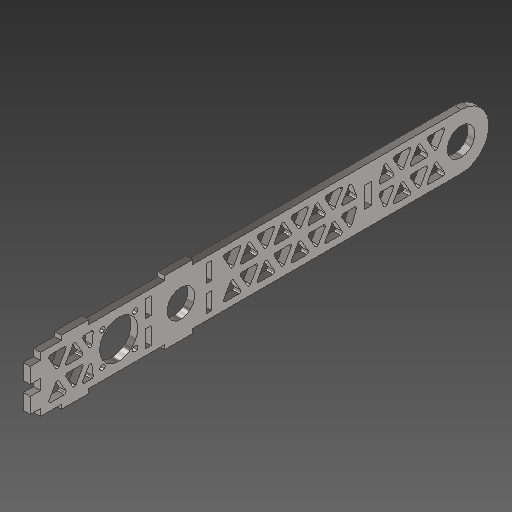
# Autodesk Inventor part: NeckFrame_02
Saved by Autodesk Inventor 2021 (Build 250183000, 183)
## iProperties
Created: 2021-03-08
Part Number: NeckFrame_02
Material: Steel, High Strength, Low Alloy
Document SubType Name: Modeling
Designer: M3rob
Density: 7.85 g/cm^3
Appearance: Steel - Polished
Mass: 5898.96 g
Surface Area: 1928.08 cm^2
Volume: 751.46 cm^3
Author: M3rob
Autodesk Inventor part; units mm, degrees
ref_plane "YZ Plane" through (0, 0, 0) normal (1, 0, 0) x (0, 1, 0)
ref_plane "XZ Plane" through (0, 0, 0) normal (0, 1, 0) x (-1, 0, 0)
ref_plane "XY Plane" through (0, 0, 0) normal (0, 0, 1) x (1, 0, 0)
sketch "Sketch1" plane through (0, 0, 0) normal (1, 0, 0) x (0, 1, 0)
  line L0 (50.8, 410.849) -> (38.1, 410.849)
  line L1 (-50.8, 410.849) -> (-50.8, 372.749)
  arc A0 (-50.8, -360.049) -> (50.8, -360.049) centre (0, -360.049) ccw
  line L2 (50.8, -360.049) -> (50.8, 132.084)
  line L3 (50.8, -360.049) -> (50.8, -410.849) construction
  line L4 (50.8, -410.849) -> (-50.8, -410.849) construction
  line L5 (-50.8, -410.849) -> (-50.8, -360.049) construction
  line L6 (0, 410.849) -> (0, -410.849) construction
  line L7 (38.1, 410.849) -> (38.1, 429.899)
  line L8 (38.1, 429.899) -> (9.525, 429.899)
  line L9 (9.525, 429.899) -> (9.525, 410.849)
  line L10 (-9.525, 410.849) -> (-9.525, 429.899)
  line L11 (-9.525, 429.899) -> (-38.1, 429.899)
  line L12 (-38.1, 429.899) -> (-38.1, 410.849)
  line L13 (9.525, 410.849) -> (-9.525, 410.849)
  line L14 (38.1, 410.849) -> (9.525, 410.849) construction
  line L15 (-9.525, 410.849) -> (-38.1, 410.849) construction
  line L16 (-38.1, 410.849) -> (-50.8, 410.849)
  line L17 (39.6875, 106.684) -> (7.9375, 106.684)
  line L18 (7.9375, 106.684) -> (7.9375, 97.159)
  line L19 (7.9375, 97.159) -> (39.6875, 97.159)
  line L20 (39.6875, 97.159) -> (39.6875, 106.684)
  line L21 (39.6875, 106.684) -> (7.9375, 97.159) construction
  line L22 (7.9375, 106.684) -> (39.6875, 97.159) construction
  line L23 (-39.6875, 106.684) -> (-7.9375, 106.684)
  line L24 (-7.9375, 106.684) -> (-7.9375, 97.159)
  line L25 (-7.9375, 97.159) -> (-39.6875, 97.159)
  line L26 (-39.6875, 97.159) -> (-39.6875, 106.684)
  line L27 (-39.6875, 106.684) -> (-7.9375, 97.159) construction
  line L28 (-7.9375, 106.684) -> (-39.6875, 97.159) construction
  line L29 (50.8, 372.749) -> (58.7375, 372.749)
  line L30 (58.7375, 372.749) -> (58.7375, 321.949)
  line L31 (58.7375, 321.949) -> (50.8, 321.949)
  line L32 (50.8, 182.884) -> (58.7375, 182.884)
  line L33 (58.7375, 182.884) -> (58.7375, 132.084)
  line L34 (58.7375, 132.084) -> (50.8, 132.084)
  line L35 (-50.8, 132.084) -> (-58.7375, 132.084)
  line L36 (-58.7375, 132.084) -> (-58.7375, 182.884)
  line L37 (-58.7375, 182.884) -> (-50.8, 182.884)
  line L38 (7.9375, 217.809) -> (39.6875, 217.809)
  line L39 (39.6875, 217.809) -> (39.6875, 208.284)
  line L40 (39.6875, 208.284) -> (7.9375, 208.284)
  line L41 (7.9375, 208.284) -> (7.9375, 217.809)
  line L42 (7.9375, 217.809) -> (39.6875, 208.284) construction
  line L43 (39.6875, 217.809) -> (7.9375, 208.284) construction
  line L44 (-39.6875, 217.809) -> (-7.9375, 217.809)
  line L45 (-7.9375, 217.809) -> (-7.9375, 208.284)
  line L46 (-7.9375, 208.284) -> (-39.6875, 208.284)
  line L47 (-39.6875, 208.284) -> (-39.6875, 217.809)
  line L48 (-39.6875, 217.809) -> (-7.9375, 208.284) construction
  line L49 (-7.9375, 217.809) -> (-39.6875, 208.284) construction
  line L50 (23.8125, 213.0465) -> (23.8125, 101.9215) construction
  line L51 (-50.8, 372.749) -> (-58.7375, 372.749)
  line L52 (-58.7375, 372.749) -> (-58.7375, 321.949)
  line L53 (-58.7375, 321.949) -> (-50.8, 321.949)
  line L54 (50.8, 321.949) -> (50.8, 372.749) construction
  line L55 (50.8, 372.749) -> (50.8, 410.849) construction
  line L56 (-50.8, 321.949) -> (-50.8, 398.5427)
  line L57 (-50.8, 372.749) -> (-50.8, 321.949) construction
  line L58 (-50.8, 182.884) -> (-50.8, 132.084) construction
  line L59 (-50.8, 132.084) -> (-50.8, -360.049)
  line L60 (50.8, 182.884) -> (50.8, 385.0553)
  line L61 (50.8, 132.084) -> (50.8, 182.884) construction
  line L62 (50.8, 398.5427) -> (41.275, 398.5427)
  line L63 (41.275, 398.5427) -> (41.275, 401.324)
  line L64 (41.275, 401.324) -> (33.3375, 401.324)
  line L65 (33.3375, 401.324) -> (33.3375, 398.5427)
  line L66 (33.3375, 398.5427) -> (30.1625, 398.5427)
  line L67 (30.1625, 398.5427) -> (30.1625, 385.0553)
  line L68 (30.1625, 385.0553) -> (33.3375, 385.0553)
  line L69 (33.3375, 385.0553) -> (33.3375, 382.274)
  line L70 (33.3375, 382.274) -> (41.275, 382.274)
  line L71 (41.275, 382.274) -> (41.275, 385.0553)
  line L72 (41.275, 385.0553) -> (50.8, 385.0553)
  line L73 (30.1625, 391.799) -> (50.8, 391.799) construction
  line L74 (-50.8, 398.5427) -> (-41.275, 398.5427)
  line L75 (-41.275, 398.5427) -> (-41.275, 401.324)
  line L76 (-41.275, 401.324) -> (-33.3375, 401.324)
  line L77 (-33.3375, 401.324) -> (-33.3375, 398.5427)
  line L78 (-33.3375, 398.5427) -> (-30.1625, 398.5427)
  line L79 (-30.1625, 398.5427) -> (-30.1625, 385.0553)
  line L80 (-30.1625, 385.0553) -> (-33.3375, 385.0553)
  line L81 (-33.3375, 385.0553) -> (-33.3375, 382.274)
  line L82 (-33.3375, 382.274) -> (-41.275, 382.274)
  line L83 (-41.275, 382.274) -> (-41.275, 385.0553)
  line L84 (-50.8, 385.0553) -> (-41.275, 385.0553)
  line L85 (50.8, 398.5427) -> (50.8, 321.949) construction
  line L86 (50.8, 385.0553) -> (50.8, 398.5427)
  line L87 (-50.8, 385.0553) -> (-50.8, 182.884)
  line L88 (-50.8, 398.5427) -> (-50.8, 385.0553) construction
  circle A1 centre (0, 267.339) radius 35.052
  circle A2 centre (0, 153.492) radius 25.4
  line L89 (50.8, 398.5427) -> (50.8, 410.849)
  line L90 (50.8, 385.0553) -> (50.8, 372.749)
  arc A3 (-32.4225, 153.492) -> (32.4225, 153.492) centre (0, 153.492) ccw
  circle A4 centre (0, -360.049) radius 25.4
  arc A5 (-62.6143, -356.6081) -> (62.6143, -356.6081) centre (0, -360.049) ccw
  point P0 (0, 0)
  point P1 (0, 0)
  point P2 (-23.8125, 101.9215)
  point P3 (23.8125, 213.0465)
  point P4 (-23.8125, 213.0465)
  point P5 (23.8125, 429.899)
  point P6 (58.7375, 157.484)
  point P7 (23.8125, 157.484)
  point P8 (23.8125, 391.799)
  point P9 (-30.1625, 391.799)
  point P10 (-50.8, 372.749)
  point P11 (-50.8, 372.749)
  dimension "d0" = 101.6
  dimension "d3" = 19.05
  dimension "d4" = 12.7
  dimension "d5" = 19.05
  dimension "d6" = 9.525
  dimension "d8" = 7.9375
  dimension "d9" = 50.8
  dimension "d12" = 31.75
  dimension "d13" = 38.1
  dimension "d14" = 9.525
  dimension "d15" = 7.9375
  dimension "d16" = 3.175
  dimension "d17" = 19.05
  dimension "d18" = 13.4874
  dimension "d23" = 143.51
  dimension "d24" = 70.104
  dimension "d25" = 50.8
  dimension "d26" = 19.05
  dimension "d39" = 50.8
  dimension "d86" = 101.6
  dimension "d92" = 193.04
  constraints: 182 end point, 100 perpendicular, 32 point on line, 18 midpoint, 15 equal length, 15 tangent, 14 horizontal, 10 vertical, 9 parallel, 6 centre point, 6 point on circle, 5 horizontal alignment, 3 concentric, 3 vertical alignment, 1 coincident, 1 collinear, 15 other
  measures "d0" distance of L0.start L1.start
  measures "d3" diameter of L9 L6
  measures "d4" distance from line of L0.start L7
  measures "d5" distance of L0.end L7.end
  measures "d6" distance of L19.end L17.start
  measures "d8" distance of L33.end L2.end
  measures "d9" distance of L32.end L33.end
  measures "d12" distance of L18.end L19.end
  measures "d13" distance from line of L29 L0.start
  measures "d14" distance of L71.end L60.end
  measures "d15" distance of L69.end L70.end
  measures "d16" distance of L67.end L68.end
  measures "d17" distance of L69.end L64.end
  measures "d18" distance between parallel lines of L72 L62
  measures "d23" distance from line of L14 A1.centre
  measures "d24" diameter of A1
  measures "d25" diameter of A2
  measures "d26" distance from line of L0 L73.end
  measures "d39" diameter of A4
  measures "d86" distance between parallel lines of L40 L17
  measures "d92" distance between parallel lines of L38 L0
extrude "Extrusion1" add sketch "Sketch1" along normal mid plane 12.7
sketch "Sketch3" plane through (6.35, 0, 0) normal (1, 0, 0) x (0, 0, -1)
  circle A0 centre (-267.339, 0) radius 34.925 construction
  line L0 (-224.159, 43.18) -> (-310.519, 43.18) construction
  line L1 (-310.519, 43.18) -> (-267.339, 0) construction
  line L2 (-310.519, -43.18) -> (-224.159, -43.18) construction
  line L3 (-267.339, 0) -> (-224.159, -43.18) construction
  line L4 (-224.159, -43.18) -> (-224.159, 43.18) construction
  line L5 (-224.159, 43.18) -> (-267.339, 0) construction
  line L6 (-310.519, 43.18) -> (-310.519, -43.18) construction
  line L7 (-267.339, 0) -> (-310.519, -43.18) construction
  circle A1 centre (-297.1803, 29.8414) radius 7.2771 construction
  circle A2 centre (-297.1803, -29.8414) radius 7.2771 construction
  circle A3 centre (-237.4976, -29.8414) radius 7.2771 construction
  circle A4 centre (-237.4976, 29.8414) radius 7.2771 construction
  circle A5 centre (-267.339, 25.019) radius 2.3813
  circle A6 centre (-292.358, 0) radius 2.3813
  circle A7 centre (-267.339, -25.019) radius 2.3813
  circle A8 centre (-242.32, 0) radius 2.3813
  circle A9 centre (-267.339, 0) radius 17.5768
  circle A10 centre (-267.339, 0) radius 35.052 projected
  dimension "d29" = 69.85
  dimension "d30" = 14.5542
  dimension "d31" = 360
  constraints: 16 end point, 10 centre point, 5 coincident, 2 collinear, 2 point on line, 1 perpendicular, 1 tangent, 13 other
  measures "d29" diameter of A0
  measures "d30" diameter of A1
hole "Hole1" at (6.35, 29.8414, 297.1803) at (6.35, 29.8414, 237.4976) at (6.35, -29.8414, 237.4976) at (6.35, -29.8414, 297.1803) direction (-1, 0, 0) diameter 9.779 end through all
sketch "Sketch4" plane through (6.35, 0, 0) normal (1, 0, 0) x (0, 0, -1)
  circle A0 centre (-358.4422, -15.0646) radius 101.6
  circle A1 centre (360.049, 0) radius 25.4
  line L0 (-90.809, 4.7625) -> (-90.809, 36.5125)
  circle A2 centre (360.049, 0) radius 406.4
  line L1 (-399.5955, -107.9568) -> (195.4357, -371.5689)
  line L2 (195.4357, -371.5689) -> (195.4357, 371.5689)
  line L3 (-65.409, -68.2625) -> (-65.409, 65.0875)
  circle A3 centre (360.049, 0) radius 25.4 projected
  line L4 (195.4357, 0) -> (182.7357, 0)
  line L5 (182.7357, 0) -> (182.7357, 19.05)
  line L6 (182.7357, 19.05) -> (195.4357, 19.05)
  line L7 (195.4357, 19.05) -> (195.4357, 0)
  line L8 (195.4357, 0) -> (182.7357, 0)
  line L9 (182.7357, 0) -> (182.7357, -19.05)
  line L10 (182.7357, -19.05) -> (195.4357, -19.05)
  line L11 (195.4357, -19.05) -> (195.4357, 0)
  point P0 (0, 0)
  point P1 (195.4357, -19.05)
  point P2 (195.4357, 19.05)
  dimension "d40" = 812.8
  dimension "d41" = 12.7
  dimension "d42" = 19.05
  dimension "d43" = 12.7
  dimension "d44" = 19.05
  dimension "d47" = 164.6133
  constraints: 24 end point, 5 parallel, 2 centre point, 2 coincident, 2 horizontal, 2 perpendicular, 2 point on circle, 1 midpoint, 1 tangent, 1 vertical, 4 other
  measures "d40" diameter of A2
  measures "d41" distance of L5.end L6.end
  measures "d42" distance of L4.end L5.end
  measures "d43" distance of L10.end L9.end
  measures "d44" distance of L9.end L8.end
  measures "d47" distance of A1.centre L4.start
extrude "Extrusion2" cut sketch "Sketch4" against normal through all contours L10 L9 L4 L2 | L2 L4 L5 L6
sketch "Sketch5" plane through (6.35, 0, 0) normal (1, 0, 0) x (0, 0, -1)
  line L0 (195.4357, -19.05) -> (182.7357, -19.05) construction
  line L1 (182.7357, -19.05) -> (182.7357, 19.05) construction
  line L2 (182.7357, 19.05) -> (195.4357, 19.05) construction
  line L3 (195.4357, 19.05) -> (195.4357, -19.05) construction
  circle A0 centre (-237.4976, -29.8414) radius 4.8895 construction
  circle A1 centre (-297.1803, 29.8414) radius 4.8895 construction
  circle A2 centre (-237.4976, 29.8414) radius 4.8895 construction
  circle A3 centre (-297.1803, -29.8414) radius 4.8895 construction
  line L4 (-410.849, -50.8) -> (-372.749, -50.8) construction
  line L5 (-372.749, -50.8) -> (-372.749, -58.7375) construction
  line L6 (-372.749, -58.7375) -> (-321.949, -58.7375) construction
  line L7 (-321.949, -58.7375) -> (-321.949, -50.8) construction
  line L8 (-321.949, -50.8) -> (-182.884, -50.8) construction
  line L9 (-182.884, -50.8) -> (-182.884, -58.7375) construction
  line L10 (-182.884, -58.7375) -> (-132.084, -58.7375) construction
  line L11 (-132.084, -58.7375) -> (-132.084, -50.8) construction
  line L12 (-132.084, -50.8) -> (360.049, -50.8) construction
  arc A4 (360.049, -50.8) -> (360.049, 50.8) centre (360.049, 0) ccw construction
  line L13 (360.049, 50.8) -> (-132.084, 50.8) construction
  line L14 (-132.084, 50.8) -> (-132.084, 58.7375) construction
  line L15 (-132.084, 58.7375) -> (-182.884, 58.7375) construction
  line L16 (-182.884, 58.7375) -> (-182.884, 50.8) construction
  line L17 (-182.884, 50.8) -> (-321.949, 50.8) construction
  line L18 (-321.949, 50.8) -> (-321.949, 58.7375) construction
  line L19 (-321.949, 58.7375) -> (-372.749, 58.7375) construction
  line L20 (-372.749, 58.7375) -> (-372.749, 50.8) construction
  line L21 (-372.749, 50.8) -> (-410.849, 50.8) construction
  line L22 (-410.849, 50.8) -> (-410.849, 38.1) construction
  line L23 (-410.849, 38.1) -> (-429.899, 38.1) construction
  line L24 (-429.899, 38.1) -> (-429.899, 9.525) construction
  line L25 (-429.899, 9.525) -> (-410.849, 9.525) construction
  line L26 (-410.849, 9.525) -> (-410.849, -9.525) construction
  line L27 (-410.849, -9.525) -> (-429.899, -9.525) construction
  line L28 (-429.899, -9.525) -> (-429.899, -38.1) construction
  line L29 (-429.899, -38.1) -> (-410.849, -38.1) construction
  line L30 (-410.849, -38.1) -> (-410.849, -50.8) construction
  circle A5 centre (-267.339, 0) radius 35.052 construction
  circle A6 centre (360.049, 0) radius 25.4 construction
  circle A7 centre (-153.492, 0) radius 25.4 construction
  line L31 (-217.809, -39.6875) -> (-217.809, -7.9375) construction
  line L32 (-217.809, -7.9375) -> (-208.284, -7.9375) construction
  line L33 (-208.284, -7.9375) -> (-208.284, -39.6875) construction
  line L34 (-208.284, -39.6875) -> (-217.809, -39.6875) construction
  line L35 (-217.809, 7.9375) -> (-217.809, 39.6875) construction
  line L36 (-217.809, 39.6875) -> (-208.284, 39.6875) construction
  line L37 (-208.284, 39.6875) -> (-208.284, 7.9375) construction
  line L38 (-208.284, 7.9375) -> (-217.809, 7.9375) construction
  line L39 (-106.684, -39.6875) -> (-106.684, -7.9375) construction
  line L40 (-106.684, -7.9375) -> (-97.159, -7.9375) construction
  line L41 (-97.159, -7.9375) -> (-97.159, -39.6875) construction
  line L42 (-97.159, -39.6875) -> (-106.684, -39.6875) construction
  line L43 (-106.684, 39.6875) -> (-97.159, 39.6875) construction
  line L44 (-97.159, 39.6875) -> (-97.159, 7.9375) construction
  line L45 (-97.159, 7.9375) -> (-106.684, 7.9375) construction
  line L46 (-106.684, 7.9375) -> (-106.684, 39.6875) construction
  line L47 (-140.0215, 38.1) -> (360.049, 38.1) construction
  arc A8 (360.049, -38.1) -> (360.049, 38.1) centre (360.049, 0) ccw construction
  line L48 (360.049, -38.1) -> (-140.0215, -38.1) construction
  line L49 (-140.0215, -38.1) -> (-140.0215, -46.0375) construction
  line L50 (-140.0215, -46.0375) -> (-165.4215, -46.0375) construction
  line L51 (-165.4215, -46.0375) -> (-165.4215, -38.1) construction
  line L52 (-165.4215, -38.1) -> (-334.649, -38.1) construction
  line L53 (-334.649, -38.1) -> (-334.649, -46.0375) construction
  line L54 (-334.649, -46.0375) -> (-360.049, -46.0375) construction
  line L55 (-360.049, -46.0375) -> (-360.049, -38.1) construction
  line L56 (-360.049, -38.1) -> (-398.149, -38.1) construction
  line L57 (-398.149, -38.1) -> (-398.149, -25.4) construction
  line L58 (-398.149, -25.4) -> (-423.549, -25.4) construction
  line L59 (-423.549, -25.4) -> (-423.549, -22.225) construction
  line L60 (-423.549, -22.225) -> (-398.149, -22.225) construction
  line L61 (-398.149, -22.225) -> (-398.149, 22.225) construction
  line L62 (-398.149, 22.225) -> (-423.549, 22.225) construction
  line L63 (-423.549, 22.225) -> (-423.549, 25.4) construction
  line L64 (-423.549, 25.4) -> (-398.149, 25.4) construction
  line L65 (-398.149, 25.4) -> (-398.149, 38.1) construction
  line L66 (-398.149, 38.1) -> (-360.049, 38.1) construction
  line L67 (-360.049, 38.1) -> (-360.049, 46.0375) construction
  line L68 (-360.049, 46.0375) -> (-334.649, 46.0375) construction
  line L69 (-334.649, 46.0375) -> (-334.649, 38.1) construction
  line L70 (-334.649, 38.1) -> (-165.4215, 38.1) construction
  line L71 (-165.4215, 38.1) -> (-165.4215, 46.0375) construction
  line L72 (-165.4215, 46.0375) -> (-140.0215, 46.0375) construction
  line L73 (-140.0215, 46.0375) -> (-140.0215, 38.1) construction
  line L74 (-398.149, 38.1) -> (-398.149, -38.1)
  line L75 (-398.149, 38.1) -> (-398.149, 0) construction
  line L76 (-398.149, 0) -> (-398.149, 6.35)
  line L77 (-398.149, 0) -> (-398.149, -6.35)
  line L78 (-398.149, 38.1) -> (-366.399, 38.1) construction
  line L79 (-398.149, 6.35) -> (-301.811, 6.35)
  circle A9 centre (-267.339, 0) radius 35.052 projected
  line L80 (-398.149, -6.35) -> (-301.811, -6.35)
  line L81 (-398.149, 38.1) -> (-379.8181, 6.35)
  line L82 (-398.149, 38.1) -> (-361.4872, 38.1) construction
  line L83 (-398.149, 38.1) -> (-361.4872, 38.1)
  line L84 (-361.4872, 38.1) -> (-379.8181, 6.35)
  line L85 (-361.4872, 38.1) -> (-348.7872, 38.1) construction
  line L86 (-348.7872, 38.1) -> (-367.1181, 6.35)
  line L87 (-348.7872, 38.1) -> (-330.4563, 6.35)
  line L88 (-330.4563, 6.35) -> (-367.1181, 6.35)
  circle A10 centre (-297.1803, 29.8414) radius 4.8895 projected
  line L89 (-302.0698, 29.8414) -> (-314.7698, 29.8414) construction
  line L90 (-348.7872, 38.1) -> (-336.0872, 38.1) construction
  line L91 (-336.0872, 38.1) -> (-317.7563, 6.35)
  line L92 (-317.7563, 6.35) -> (-313.8951, 38.1)
  circle A11 centre (-297.1803, 29.8414) radius 17.5895 construction
  line L93 (-313.8951, 38.1) -> (-336.0872, 38.1)
  line L94 (-398.149, 0) -> (-389.5764, 0)
  line L95 (-398.149, -38.1) -> (-379.8181, -6.35)
  line L96 (-398.149, -38.1) -> (-361.4872, -38.1)
  line L97 (-361.4872, -38.1) -> (-379.8181, -6.35)
  line L98 (-348.7872, -38.1) -> (-367.1181, -6.35)
  line L99 (-348.7872, -38.1) -> (-330.4563, -6.35)
  line L100 (-330.4563, -6.35) -> (-367.1181, -6.35)
  line L101 (-336.0872, -38.1) -> (-317.7563, -6.35)
  line L102 (-317.7563, -6.35) -> (-313.8951, -38.1)
  line L103 (-313.8951, -38.1) -> (-336.0872, -38.1)
  line L104 (-97.159, 39.6875) -> (-97.159, 7.9375) projected
  line L105 (-92.3965, 38.1) -> (-79.6965, 38.1) construction
  line L106 (-41.4472, 38.1) -> (-59.7781, 6.35)
  line L107 (-78.109, 38.1) -> (-41.4472, 38.1)
  line L108 (-78.109, 38.1) -> (-59.7781, 6.35)
  line L109 (-41.4472, -38.1) -> (-59.7781, -6.35)
  line L110 (-78.109, -38.1) -> (-41.4472, -38.1)
  line L111 (-78.109, -38.1) -> (-59.7781, -6.35)
  line L112 (-28.7472, -38.1) -> (-47.0781, -6.35)
  line L113 (-28.7472, -38.1) -> (-10.4163, -6.35)
  line L114 (-10.4163, -6.35) -> (-47.0781, -6.35)
  line L115 (-28.7472, 38.1) -> (-10.4163, 6.35)
  line L116 (-10.4163, 6.35) -> (-47.0781, 6.35)
  line L117 (-28.7472, 38.1) -> (-47.0781, 6.35)
  line L118 (20.605, 38.1) -> (2.2741, 6.35)
  line L119 (20.605, -38.1) -> (2.2741, -6.35)
  line L120 (-16.0568, 38.1) -> (2.2741, 6.35)
  line L121 (-16.0568, -38.1) -> (2.2741, -6.35)
  line L122 (33.305, -38.1) -> (14.9741, -6.35)
  line L123 (33.305, 38.1) -> (14.9741, 6.35)
  line L124 (33.305, -38.1) -> (51.6359, -6.35)
  line L125 (33.305, 38.1) -> (51.6359, 6.35)
  line L126 (51.6359, 6.35) -> (14.9741, 6.35)
  line L127 (51.6359, -6.35) -> (14.9741, -6.35)
  line L128 (-16.0568, 38.1) -> (20.605, 38.1)
  line L129 (-16.0568, -38.1) -> (20.605, -38.1)
  line L130 (82.6572, 38.1) -> (64.3263, 6.35)
  line L131 (82.6572, -38.1) -> (64.3263, -6.35)
  line L132 (45.9954, 38.1) -> (64.3263, 6.35)
  line L133 (45.9954, -38.1) -> (64.3263, -6.35)
  line L134 (95.3572, -38.1) -> (77.0263, -6.35)
  line L135 (95.3572, 38.1) -> (77.0263, 6.35)
  line L136 (95.3572, -38.1) -> (113.6881, -6.35)
  line L137 (95.3572, 38.1) -> (113.6881, 6.35)
  line L138 (113.6881, 6.35) -> (77.0263, 6.35)
  line L139 (113.6881, -6.35) -> (77.0263, -6.35)
  line L140 (45.9954, 38.1) -> (82.6572, 38.1)
  line L141 (45.9954, -38.1) -> (82.6572, -38.1)
  line L142 (144.7094, 38.1) -> (126.3785, 6.35)
  line L143 (144.7094, -38.1) -> (126.3785, -6.35)
  line L144 (108.0476, 38.1) -> (126.3785, 6.35)
  line L145 (108.0476, -38.1) -> (126.3785, -6.35)
  line L146 (157.4094, -38.1) -> (139.0785, -6.35)
  line L147 (157.4094, 38.1) -> (139.0785, 6.35)
  line L148 (157.4094, -38.1) -> (175.7403, -6.35)
  line L149 (157.4094, 38.1) -> (175.7403, 6.35)
  line L150 (175.7403, 6.35) -> (139.0785, 6.35)
  line L151 (175.7403, -6.35) -> (139.0785, -6.35)
  line L152 (108.0476, 38.1) -> (144.7094, 38.1)
  line L153 (108.0476, -38.1) -> (144.7094, -38.1)
  line L154 (182.7357, -19.05) -> (182.7357, 19.05) projected
  line L155 (182.7357, 0) -> (170.0357, 0) construction
  line L156 (170.0357, 0) -> (170.0357, 6.35) construction
  line L157 (170.0357, 0) -> (170.0357, -6.35) construction
  line L158 (157.4094, -38.1) -> (170.0357, -6.35)
  line L159 (157.4094, 38.1) -> (170.0357, 6.35)
  line L160 (189.0857, -19.05) -> (189.0857, 0)
  line L161 (295.5141, 38.1) -> (313.845, 6.35)
  line L162 (295.5141, -38.1) -> (313.845, -6.35)
  line L163 (332.1759, 38.1) -> (313.845, 6.35)
  line L164 (332.1759, -38.1) -> (313.845, -6.35)
  line L165 (282.8141, -38.1) -> (301.145, -6.35)
  line L166 (282.8141, 38.1) -> (301.145, 6.35)
  line L167 (282.8141, -38.1) -> (264.4833, -6.35)
  line L168 (282.8141, 38.1) -> (264.4833, 6.35)
  line L169 (264.4833, 6.35) -> (301.145, 6.35)
  line L170 (264.4833, -6.35) -> (301.145, -6.35)
  line L171 (332.1759, 38.1) -> (295.5141, 38.1)
  line L172 (332.1759, -38.1) -> (295.5141, -38.1)
  line L173 (233.4619, 38.1) -> (251.7928, 6.35)
  line L174 (233.4619, -38.1) -> (251.7928, -6.35)
  line L175 (270.1237, 38.1) -> (251.7928, 6.35)
  line L176 (270.1237, -38.1) -> (251.7928, -6.35)
  line L177 (220.7619, -38.1) -> (239.0928, -6.35)
  line L178 (220.7619, 38.1) -> (239.0928, 6.35)
  line L179 (220.7619, -38.1) -> (202.4311, -6.35)
  line L180 (220.7619, 38.1) -> (202.4311, 6.35)
  line L181 (202.4311, 6.35) -> (239.0928, 6.35)
  line L182 (202.4311, -6.35) -> (239.0928, -6.35)
  line L183 (270.1237, 38.1) -> (233.4619, 38.1)
  line L184 (270.1237, -38.1) -> (233.4619, -38.1)
  line L185 (195.4357, 0) -> (208.1357, 0) construction
  line L186 (208.1357, 0) -> (208.1357, 6.35) construction
  line L187 (208.1357, 0) -> (208.1357, -6.35) construction
  line L188 (220.7619, -38.1) -> (208.1357, -6.35)
  line L189 (220.7619, 38.1) -> (208.1357, 6.35)
  line L190 (-106.684, 7.9375) -> (-106.684, 39.6875) projected
  line L191 (-101.9215, 38.1) -> (-114.6215, 38.1) construction
  circle A12 centre (-153.492, 0) radius 38.1
  line L192 (-106.684, 7.9375) -> (-114.6215, 7.9375)
  line L193 (-114.6215, 7.9375) -> (-114.6215, 38.1)
  line L194 (-114.6215, 38.1) -> (-101.9215, 38.1)
  line L195 (-101.9215, 38.1) -> (-101.9215, 7.9375)
  line L196 (-140.0215, 38.1) -> (-140.0215, 35.6392)
  line L197 (-114.6215, 7.9375) -> (-116.228, 7.9375)
  line L198 (-114.6215, 38.1) -> (-140.0215, 38.1)
  line L199 (-106.684, -7.9375) -> (-114.6215, -7.9375)
  line L200 (-114.6215, -7.9375) -> (-114.6215, -38.1)
  line L201 (-114.6215, -38.1) -> (-101.9215, -38.1)
  line L202 (-101.9215, -38.1) -> (-101.9215, -7.9375)
  line L203 (-114.6215, -7.9375) -> (-116.228, -7.9375)
  line L204 (-140.0215, -38.1) -> (-114.6215, -38.1)
  line L205 (-140.0215, -38.1) -> (-140.0215, -35.6392)
  line L206 (-208.284, -7.9375) -> (-190.8215, -7.9375)
  line L207 (-190.8215, -7.9375) -> (-190.8215, -38.1)
  line L208 (-190.8215, -38.1) -> (-203.5215, -38.1)
  line L209 (-203.5215, -38.1) -> (-203.5215, -7.9375)
  line L210 (-208.284, 39.6875) -> (-208.284, 7.9375) projected
  line L211 (-203.5215, 38.1) -> (-190.8215, 38.1)
  line L212 (-190.8215, 38.1) -> (-190.8215, 7.6238)
  line L213 (-190.8215, 7.6238) -> (-203.5215, 7.6238)
  line L214 (-203.5215, 7.6238) -> (-203.5215, 38.1)
  line L215 (-165.4215, 38.1) -> (-165.4215, 36.1842)
  line L216 (-165.4215, 38.1) -> (-190.8215, 38.1)
  line L217 (-190.8215, -38.1) -> (-165.4215, -38.1)
  line L218 (-165.4215, -36.1842) -> (-165.4215, -38.1)
  point P0 (0, 0)
  point P1 (-330.4563, -6.35)
  point P2 (-367.1181, -6.35)
  dimension "d48" = 12.7
  dimension "d49" = 76.2
  dimension "d50" = 38.1
  dimension "d51" = 6.35
  dimension "d52" = 6.35
  dimension "d57" = 60
  dimension "d58" = 36.6617
  dimension "d59" = 36.6617
  dimension "d60" = 12.7
  dimension "d61" = 36.6617
  dimension "d62" = 36.6617
  dimension "d63" = 12.7
  dimension "d64" = 12.7
  dimension "d65" = 36.6617
  dimension "d66" = 90
  dimension "d70" = 12.7
  dimension "d73" = 320.04
  dimension "d80" = 62.0522
  dimension "d85" = 12.7
  dimension "d87" = 12.7
  dimension "d88" = 12.7
  dimension "d89" = 12.7
  dimension "d90" = 12.7
  dimension "d91" = 12.7
  constraints: 336 end point, 36 symmetric about line, 21 point on line, 17 horizontal, 9 parallel, 8 perpendicular, 6 collinear, 4 point on circle, 3 midpoint, 3 vertical, 2 horizontal alignment, 1 centre point, 1 coincident, 1 equal length, 142 other
  measures "d48" distance between parallel lines of L13 L47
  measures "d49" distance of L65.end L56.end
  measures "d50" distance of L65.end L75.end
  measures "d51" distance of L75.end L76.end
  measures "d52" distance of L75.end L77.end
  measures "d57" angle of L81 L82
  measures "d58" distance of L65.end L81.end
  measures "d59" distance of L65.end L82.end
  measures "d60" distance of L82.end L85.end
  measures "d61" distance of L85.end L86.end
  measures "d62" distance of L85.end L87.end
  measures "d63" distance of L89.start L89.end
  measures "d64" distance of L85.end L90.end
  measures "d65" distance of L90.end L91.end
  measures "d66" angle of L61 L94
  measures "d70" distance of L105.start L105.end
  measures "d73" distance of L82.end L106.start
  measures "d80" distance of L109.end L119.end
  measures "d85" distance of L155.start L155.end
  measures "d87" distance of L191.start L191.end
  measures "d89" distance of L201.end L200.end
  measures "d90" distance of L207.end L208.end
  measures "d91" distance of L212.end L213.end
extrude "Extrusion3" cut sketch "Sketch5" against normal through all contours L83 L84 L81 | L91 L93 L92 | L102 L103 L101 | L86 L87 L79 | L95 L97 L96 | L80 L99 L98 | L106 L108 L107 | L110 L111 L109 | L112 L114 L113 | L115 L116 L117 | L118 L120 L128 | L129 L121 L119 | L122 L127 L124 | L125 L126 L123 | L130 L132 L140 | L141 L133 L131 | L134 L139 L136 | L137 L138 L135 | L142 L144 L152 | L153 L145 L143 | L146 L151 L158 | L159 L150 L147 | L171 L163 L161 | L162 L164 L172 | L167 L170 L165 | L166 L169 L168 | L183 L175 L173 | L174 L176 L184 | L188 L182 L177 | L178 L181 L189
fillet "Fillet1" radius 3.175 90 edges at (0, 38.1, 313.8951) (0, 38.1, 336.0872) (0, 38.1, 348.7872) (0, 6.35, 367.1181) (0, 6.35, 330.4563) (0, 6.35, 317.7563) (0, -38.1, 348.7872) (0, 38.1, 361.4872) (0, 38.1, 398.149) (0, 6.35, 379.8181) (0, -6.35, 367.1181) (0, -6.35, 330.4563) (0, -6.35, 379.8181) (0, -38.1, 398.149) (0, -38.1, 361.4872) (0, -38.1, 336.0872) (0, -38.1, 313.8951) (0, -6.35, 317.7563) (0, 38.1, 78.109) (0, -6.35, 59.7781) (0, 6.35, 59.7781) (0, 38.1, 41.4472) (0, 38.1, 28.7472) (0, 6.35, 10.4163) (0, 6.35, -2.2741) (0, 38.1, 16.0568) (0, 38.1, -20.605) (0, 6.35, 47.0781) (0, -38.1, 41.4472) (0, -38.1, 78.109) (0, -38.1, 28.7472) (0, -6.35, 47.0781) (0, -6.35, 10.4163) (0, -6.35, -2.2741) (0, -38.1, -20.605) (0, -38.1, 16.0568) (0, -38.1, -33.305) (0, -6.35, -14.9741) (0, -6.35, -51.6359) (0, 6.35, -51.6359) (0, 6.35, -14.9741) (0, 38.1, -33.305) (0, 38.1, -45.9954) (0, 38.1, -82.6572) (0, 6.35, -64.3263) (0, -6.35, -64.3263) (0, -38.1, -82.6572) (0, -38.1, -45.9954) (0, -38.1, -95.3572) (0, -6.35, -77.0263) (0, -6.35, -113.6881) (0, 6.35, -113.6881) (0, 6.35, -77.0263) (0, 38.1, -95.3572) (0, 38.1, -144.7094) (0, 38.1, -108.0476) (0, 6.35, -126.3785) (0, -38.1, -144.7094) (0, -38.1, -108.0476) (0, -6.35, -126.3785) (0, -38.1, -157.4094) (0, -6.35, -139.0785) (0, -6.35, -170.0357) (0, 6.35, -170.0357) (0, 6.35, -139.0785) (0, 38.1, -157.4094) (0, 38.1, -220.7619) (0, 6.35, -208.1357) (0, 6.35, -239.0928) (0, 6.35, -251.7928) (0, 38.1, -233.4619) (0, 38.1, -270.1237) (0, 38.1, -282.8141) (0, 6.35, -264.4833) (0, 6.35, -301.145) (0, 38.1, -295.5141) (0, 38.1, -332.1759) (0, 6.35, -313.845) (0, -6.35, -313.845) (0, -38.1, -332.1759) (0, -38.1, -295.5141) (0, -38.1, -282.8141) (0, -38.1, -270.1237) (0, -38.1, -233.4619) (0, -38.1, -220.7619) (0, -6.35, -208.1357) (0, -6.35, -239.0928) (0, -6.35, -251.7928) (0, -6.35, -264.4833) (0, -6.35, -301.145)
equation "\"d26\" = 0.5 * d13"
body "Solid1"
